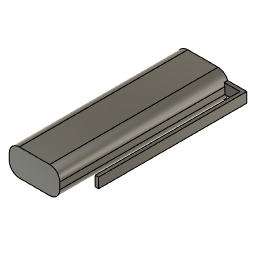
Pico Bot v15 (Autodesk Fusion 360 archive; units mm, degrees)
design "Lipo small long"
Autodesk Fusion 360 part; units mm, degrees
sketch "Sketch1" plane through (0, 0, 0) normal (0, 0, 1) x (1, 0, 0)
  line L0 (-7.5, 25) -> (7.5, 25)
  line L1 (7.5, 25) -> (7.5, -25)
  line L2 (7.5, -25) -> (-7.5, -25)
  line L3 (-7.5, -25) -> (-7.5, 25)
  line L4 (0, 0) -> (25, 0) construction
  line L5 (0, 0) -> (0, 25) construction
  line L6 (7.5, 25) -> (13, 25)
  line L7 (13, 25) -> (13, -19)
  line L8 (13, -19) -> (12, -19)
  line L9 (12, -19) -> (12, 24)
  line L10 (12, 24) -> (7.5, 24)
  dimension "d1" = 15
  dimension "d2" = 50
  constraint horizontal L0
  constraint vertical L1
  constraint horizontal L2
  constraint vertical L3
  constraint coincident L4.start L5.start
  constraint perpendicular L1 L4
  constraint perpendicular L4 L5
  constraint symmetric L1 L3 L5
  constraint symmetric L0 L2 L4
  constraint perpendicular L1 L6
  constraint perpendicular L4 L7
  constraint perpendicular L7 L8
  constraint perpendicular L4 L9
  constraint coincident L1 L10.end
  constraint perpendicular L1 L10
  measures "d1" distance of L0.start L0.end
  measures "d2" distance of L0.start L2.end
extrude "Extrude1" add sketch "Sketch1" along normal blind 8 contours L0 L1 L2 L3
extrude "Extrude2" add sketch "Sketch1" along normal blind 3 from surface at 3 contours L1 L6 L7 L8 L9 L10
fillet "Fillet1" radius 3 4 edges at (-7.5, 0, 8) (7.5, 0, 8) (7.5, 0, 0) (-7.5, 0, 0)

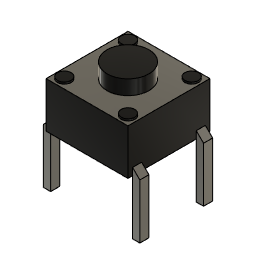
design "Button - 4.5mm x 4.5mm"
Autodesk Fusion 360 part; units mm, degrees
sketch "Sketch1" plane through (0, 0, 0) normal (0, 0, 1) x (1, 0, 0)
  line L0 (-2.25, 2.25) -> (2.25, 2.25)
  line L1 (2.25, 2.25) -> (2.25, -2.25)
  line L2 (2.25, -2.25) -> (-2.25, -2.25)
  line L3 (-2.25, -2.25) -> (-2.25, 2.25)
  line L4 (0, 0) -> (7.5, 0) construction
  line L5 (0, 0) -> (0, 6.7508) construction
  circle A0 centre (0, 0) radius 1.15
  circle A1 centre (-1.75, -1.75) radius 0.375
  circle A2 centre (1.75, -1.75) radius 0.375
  circle A3 centre (1.75, 1.75) radius 0.375
  circle A4 centre (-1.75, 1.75) radius 0.375
  line L6 (-2.25, -1.5) -> (-2.65, -1.5)
  line L7 (-2.65, -1.5) -> (-2.65, -2)
  line L8 (-2.65, -2) -> (-2.25, -2)
  line L9 (-2.25, -2) -> (-2.25, -1.5)
  line L10 (-2.25, 2) -> (-2.25, 1.5)
  line L11 (-2.65, 2) -> (-2.25, 2)
  line L12 (-2.65, 1.5) -> (-2.65, 2)
  line L13 (-2.25, 1.5) -> (-2.65, 1.5)
  line L14 (2.65, 2) -> (2.25, 2)
  line L15 (2.65, 1.5) -> (2.65, 2)
  line L16 (2.25, 1.5) -> (2.65, 1.5)
  line L17 (2.25, 2) -> (2.25, 1.5)
  line L18 (2.25, -2) -> (2.25, -1.5)
  line L19 (2.25, -1.5) -> (2.65, -1.5)
  line L20 (2.65, -1.5) -> (2.65, -2)
  line L21 (2.65, -2) -> (2.25, -2)
  dimension "d3" = 4.5
  dimension "d4" = 4.5
  dimension "d5" = 2.3
  dimension "d6" = 0.75
  dimension "d7" = 1.75
  dimension "d8" = 1.75
  dimension "d10" = 360
  dimension "d11" = 0.4
  dimension "d12" = 0.5
  dimension "d13" = 0.25
  constraint horizontal L0
  constraint vertical L1
  constraint horizontal L2
  constraint vertical L3
  constraint coincident L4.start L5.start
  constraint horizontal L4
  constraint perpendicular L4 L5
  constraint symmetric L1 L3 L5
  constraint symmetric L0 L2 L4
  constraint horizontal L6
  constraint vertical L7
  constraint horizontal L8
  constraint vertical L9
  constraint collinear L3 L9
  constraint symmetric L4 L6.start L10.end
  constraint symmetric L4 L6.end L12.start
  constraint symmetric L4 L7.end L11.start
  constraint symmetric L4 L8.end L10.start
  constraint symmetric L5 L6.start L18.end
  constraint symmetric L5 L6.end L19.end
  constraint symmetric L5 L7.end L20.end
  constraint symmetric L5 L8.end L18.start
  constraint symmetric L5 L10.start L14.end
  constraint symmetric L5 L10.end L16.start
  constraint symmetric L5 L11.start L14.start
  constraint symmetric L5 L12.start L15.start
  measures "d3" distance of L0.start L0.end
  measures "d4" distance of L0.start L2.end
  measures "d5" diameter of A0
  measures "d6" diameter of A1
  measures "d7" horizontal distance of L4.start A1.centre
  measures "d8" vertical distance of L4.start A1.centre
  measures "d11" distance of L7 L9
  measures "d12" distance of L6 L8
  measures "d13" distance of L2 L8
extrude "Extrude1" add sketch "Sketch1" along normal blind 2.5 contours L0 L1 L2 L3 L9 L10 L17 L18 | A0 | A1 | A2 | A3 | A4
extrude "Extrude2" add sketch "Sketch1" along normal blind -3 and the other way blind -0.4 contours L3 L10 L11 L12 L13 | L1 L14 L15 L16 L17 | L3 L6 L7 L8 L9 | L1 L18 L19 L20 L21
chamfer "Chamfer1" distance 0.4 angle 45 4 edges at (2.65, -1.75, 0.4) (2.65, 1.75, 0.4) (-2.65, 1.75, 0.4) (-2.65, -1.75, 0.4)
extrude "Extrude3" add sketch "Sketch1" along normal blind 0.1 from surface at 2.5 contours A1 | A2 | A3 | A4
extrude "Extrude4" add sketch "Sketch1" along normal blind 0.8 from surface at 2.5 contours A0
